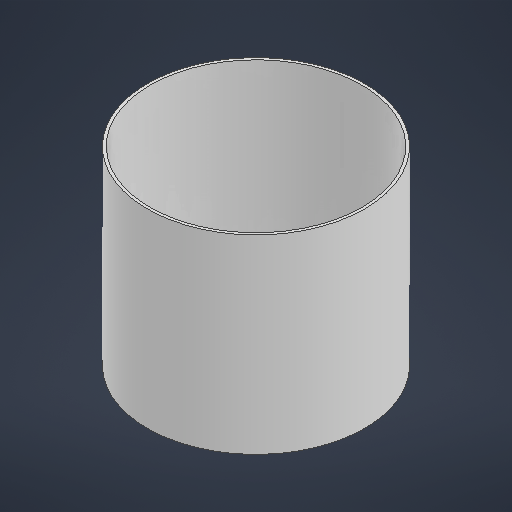
# Autodesk Inventor part: Bin
Saved by Autodesk Inventor 2027 (Build 310192060, 192F)
## iProperties
Created: 2026-06-18
Part Number: Bin
Material: Generic
Document SubType Name: Modeling
Designer: 13129
Density: 1 g/cm^3
Appearance: Default
Author: 13129
Autodesk Inventor part; units mm, degrees
ref_plane "YZ Plane" through (0, 0, 0) normal (1, 0, 0) x (0, 1, 0)
ref_plane "XZ Plane" through (0, 0, 0) normal (0, 1, 0) x (-1, 0, 0)
ref_plane "XY Plane" through (0, 0, 0) normal (0, 0, 1) x (1, 0, 0)
sketch "Sketch1" plane through (0, 0, 0) normal (0, 1, 0) x (-1, 0, 0)
  circle A0 centre (0, 0) radius 152.4
  dimension "d0" = 304.8
  constraints: 1 centre point, 1 coincident
  measures "d0" diameter of A0
extrude "Extrusion1" add sketch "Sketch1" along normal blind 12.7
sketch "Sketch2" plane through (0, 12.7, 0) normal (0, 1, 0) x (1, 0, 0)
  circle A0 centre (0, 0) radius 152.4 construction
  circle A1 centre (0, 0) radius 152.4
  circle A2 centre (0, 0) radius 148.59
  dimension "d3" = 297.18
  constraints: 2 centre point, 2 coincident, 1 concentric
  measures "d3" diameter of A2
extrude "Extrusion2" add sketch "Sketch2" along normal blind 254
body "Solid1"
